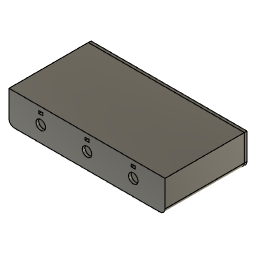
Massive Knob housing - 3 pots, under desk, Arduino Pro Micro (Autodesk Fusion 360 design; units mm, degrees)
Autodesk Fusion 360 part; units mm, degrees
sketch "Housing" plane through (0, 0, 0) normal (0, 1, 0) x (1, 0, 0) in component "Housing"
  line L0 (0, 0) -> (118, 0)
  circle A0 centre (24, -12) radius 3.6
  line L1 (24, -12) -> (24, -20.75) construction
  line L2 (25.5, -20.75) -> (22.5, -20.75)
  line L3 (22.5, -20.75) -> (22.5, -18.75)
  line L4 (22.5, -18.75) -> (25.5, -18.75)
  line L5 (25.5, -18.75) -> (25.5, -20.75)
  circle A1 centre (24, -12) radius 10 construction
  line L6 (24, -12) -> (59, -12) construction
  line L7 (59, -12) -> (94, -12) construction
  circle A2 centre (59, -12) radius 3.6
  circle A3 centre (94, -12) radius 3.6
  line L8 (57.5, -20.75) -> (60.5, -20.75)
  line L9 (60.5, -20.75) -> (60.5, -18.75)
  line L10 (60.5, -18.75) -> (57.5, -18.75)
  line L11 (57.5, -18.75) -> (57.5, -20.75)
  line L12 (92.5, -20.75) -> (95.5, -20.75)
  line L13 (95.5, -20.75) -> (95.5, -18.75)
  line L14 (95.5, -18.75) -> (92.5, -18.75)
  line L15 (92.5, -18.75) -> (92.5, -20.75)
  line L16 (59, -12) -> (59, -20.75) construction
  line L17 (94, -12) -> (94, -20.75) construction
  line L18 (24, -12) -> (24, 0) construction
  line L19 (24, -12) -> (0, -12) construction
  line L20 (94, -12) -> (118, -12) construction
  line L21 (24, -12) -> (24, -24) construction
  line L22 (0, 0) -> (0, -24)
  line L23 (0, -24) -> (118, -24)
  line L24 (118, -24) -> (118, 0)
  line L25 (2, -2) -> (116, -2)
  line L26 (116, -22) -> (116, -2)
  line L27 (2, -22) -> (116, -22)
  line L28 (2, -2) -> (2, -22)
  arc A4 (2, -18) -> (2, -6) centre (2, -12) ccw
  circle A5 centre (3.75, -12) radius 1.75
  arc A6 (116, -6) -> (116, -18) centre (116, -12) ccw
  circle A7 centre (114.25, -12) radius 1.75
  dimension "d1" = 7.2
  dimension "d2" = 8.75
  dimension "d3" = 2
  dimension "d4" = 3
  dimension "d5" = 20
  dimension "d6" = 35
  dimension "d17" = -2
  dimension "d22" = 6
  dimension "d23" = 3.5
  dimension "d24" = 6
  dimension "d25" = 3.5
  dimension "d49" = 24
  dimension "d50" = 12
  constraint coincident L0.start L22.start
  constraint horizontal L0
  constraint coincident A0.centre L1.start
  constraint vertical L1
  constraint horizontal L2
  constraint vertical L3
  constraint horizontal L4
  constraint vertical L5
  constraint midpoint L1.end L2
  constraint concentric A0 A1
  constraint perpendicular L1 L6
  constraint parallel L6 L7
  constraint coincident L6.end L7.start
  constraint coincident L7.end A3.centre
  constraint horizontal L8
  constraint vertical L9
  constraint horizontal L10
  constraint vertical L11
  constraint horizontal L12
  constraint vertical L13
  constraint horizontal L14
  constraint vertical L15
  constraint equal L2 L8
  constraint equal L3 L11
  constraint equal L2 L12
  constraint equal L3 L15
  constraint equal A0 A2
  constraint equal A0 A3
  constraint equal L6 L7
  constraint midpoint L8 L16.end
  constraint midpoint L12 L17.end
  constraint vertical L16
  constraint vertical L17
  constraint equal L1 L16
  constraint equal L1 L17
  constraint coincident L0 L18.end
  constraint perpendicular L0 L18
  constraint perpendicular L1 L19
  constraint perpendicular L17 L20
  constraint perpendicular L19 L21
  constraint perpendicular L19 L22
  constraint perpendicular L22 L23
  constraint perpendicular L0 L24
  constraint coincident L21.end L23
  constraint coincident L19.end L22
  constraint coincident L20.end L24
  constraint coincident L28 A4.end
  constraint midpoint L28 A4.centre
  constraint coincident L19 A5.centre
  constraint coincident A4.centre A5
  constraint coincident L26 A6.start
  constraint midpoint L26 A6.centre
  constraint coincident L20 A7.centre
  constraint coincident A6.centre A7
  constraint equal L19 L20
  constraint equal L18 L21
  measures "d1" diameter of A0
  measures "d2" distance of A0.centre L1.end
  measures "d3" distance of L2.start L4.end
  measures "d4" distance of L2.start L2.end
  measures "d5" diameter of A1
  measures "d6" distance of A0.centre L6.end
  measures "d22" radius of A4
  measures "d23" diameter of A5
  measures "d24" distance of A6.centre A6.start
  measures "d25" diameter of A7
  measures "d49" distance of A0.centre L19.end
  measures "d50" distance of A0.centre L21.end
extrude "Extrude1" add sketch "Housing" along normal blind 2 contours L25 L26 L27 L28 A4 A6 | A5 | L28 A4 | A7 | L26 A6 makes body 1 in component "Housing"
extrude "Extrude3" add sketch "Housing" along normal blind 60 contours L0 L22 L23 L24 bodies 1 in component "Housing"
extrude "Extrude4" add sketch "Housing" against normal blind 5 from surface at 60 contours L28 A4 | L26 A6 bodies 1 in component "Housing"
extrude "Extrude5" add sketch "Housing" against normal blind 2 from surface at 55 contours A5 | L28 A4 | A7 | L26 A6 bodies 1 in component "Housing"
fillet "Fillet1" radius 4 4 edges at (116, 31, 2) (2, 31, 2) (118, 30, 0) (0, 30, 0) on bodies 1 in component "Housing"
chamfer "Chamfer1" distance 5.99 angle 45 2 edges at (2, 53, 12) (116, 53, 12) on bodies 1 in component "Housing"
ref_plane "WorkPlane1" through (0, 60, 0) normal (0, 1, 0) x (0, 0, 1) in component "Lid"
sketch "Lid" plane through (0, 60, 0) normal (0, 1, 0) x (1, 0, 0) in component "Lid"
  arc A0 (6, -2) -> (2, -6) centre (6, -6) ccw construction
  arc A1 (2, -18) -> (2, -6) centre (2, -12) ccw construction
  line L0 (2, -22) -> (2, -18) construction
  line L1 (116, -22) -> (2, -22) construction
  line L2 (6, -2) -> (112, -2) construction
  arc A2 (116, -6) -> (112, -2) centre (112, -6) ccw construction
  arc A3 (116, -6) -> (116, -18) centre (116, -12) ccw construction
  line L3 (116, -18) -> (116, -22) construction
  circle A4 centre (114.25, -12) radius 1.75 construction
  circle A5 centre (3.75, -12) radius 1.75 construction
  circle A6 centre (114.25, -12) radius 1.5
  circle A7 centre (3.75, -12) radius 1.5
  line L4 (0, -24) -> (118, -24)
  line L5 (0, -4) -> (0, -24)
  arc A8 (4, 0) -> (0, -4) centre (4, -4) ccw
  line L6 (114, 0) -> (4, 0)
  arc A9 (118, -4) -> (114, 0) centre (114, -4) ccw
  line L7 (118, -24) -> (118, -4)
  arc A10 (6, -2.4) -> (2.4208, -5.6138) centre (6, -6) ccw
  arc A11 (2.4, -18.3875) -> (2.4208, -5.6138) centre (2, -12) ccw
  line L8 (2.4, -21.6) -> (2.4, -18.3875)
  line L9 (115.6, -21.6) -> (2.4, -21.6)
  line L10 (115.6, -18.3875) -> (115.6, -21.6)
  arc A12 (115.5792, -5.6138) -> (115.6, -18.3875) centre (116, -12) ccw
  arc A13 (115.5792, -5.6138) -> (112, -2.4) centre (112, -6) ccw
  line L11 (6, -2.4) -> (112, -2.4)
  arc A14 (6, -4.4) -> (5.6561, -4.4374) centre (6, -6) ccw
  arc A15 (5.5777, -19.6) -> (5.6561, -4.4374) centre (2, -12) ccw
  line L12 (112.4223, -19.6) -> (5.5777, -19.6)
  arc A16 (112.3439, -4.4374) -> (112.4223, -19.6) centre (116, -12) ccw
  arc A17 (112.3439, -4.4374) -> (112, -4.4) centre (112, -6) ccw
  line L13 (6, -4.4) -> (112, -4.4)
  dimension "d51" = 3
  dimension "d52" = 3
  dimension "d53" = 0.4
  dimension "d54" = 2.4
  constraint concentric A4 A6
  constraint concentric A5 A7
  measures "d51" diameter of A6
  measures "d52" diameter of A7
extrude "Extrude1'" add sketch "Lid" along normal blind 2 separate body contours L4 L5 A8 L6 A9 L7 | A10 A11 L8 L9 L10 A12 A13 L11 | A14 A15 L12 A16 A17 L13 makes body 2 in component "Lid"
extrude "Extrude2" add sketch "Lid" against normal blind 2 contours A10 A11 L8 L9 L10 A12 A13 L11 bodies 2 in component "Lid"
sketch "Arduino Pro Micro USB port" plane through (0, 0, 0) normal (-1, 0, 0) x (0, -1, 0) in component "Housing"
  line L0 (-60, 4) -> (0, 4)
  line L1 (0, 4) -> (0, 24)
  line L2 (0, 24) -> (-60, 24)
  line L3 (-60, 24) -> (-60, 4)
  line L4 (-2, 22) -> (-60, 22)
  line L5 (-31, 22) -> (-31, 19) construction
  line L6 (-35, 19) -> (-27, 19)
  line L7 (-27, 19) -> (-27, 16)
  line L8 (-27, 16) -> (-35, 16)
  line L9 (-35, 16) -> (-35, 19)
  dimension "d43" = 3
  dimension "d44" = 8
  dimension "d45" = 3
  constraint midpoint L4 L5.start
  constraint perpendicular L4 L5
  constraint horizontal L6
  constraint vertical L7
  constraint horizontal L8
  constraint vertical L9
  constraint midpoint L5.end L6
  measures "d43" distance of L5.start L5.end
  measures "d44" distance of L6.start L6.end
  measures "d45" distance of L6.start L8.end
extrude "Extrude6" cut sketch "Arduino Pro Micro USB port" against normal blind 2 contours L6 L7 L8 L9 bodies 1 in component "Housing"
chamfer "Chamfer2" distance 1 angle 45 2 edges at (1, 27, 19) (1, 35, 19) on bodies 1 in component "Housing"
sketch "Arduino Pro Micro support" plane through (0, 0, 22) normal (0, 0, -1) x (1, 0, 0) in component "Housing"
  line L0 (116, -2) -> (2, -2)
  line L1 (2, -2) -> (2, -60)
  line L2 (2, -60) -> (116, -60)
  line L3 (116, -60) -> (116, -2)
  line L4 (2, -2) -> (2, -60)
  line L5 (2, -31) -> (35.5, -31) construction
  line L6 (37.5, -36) -> (35.5, -36)
  line L7 (35.5, -36) -> (35.5, -26)
  line L8 (35.5, -26) -> (37.5, -26)
  line L9 (37.5, -26) -> (37.5, -36)
  dimension "d55" = 33.5
  dimension "d56" = 2
  dimension "d57" = 10
  constraint midpoint L4 L5.start
  constraint perpendicular L1 L5
  constraint horizontal L6
  constraint vertical L7
  constraint horizontal L8
  constraint vertical L9
  constraint midpoint L5.end L7
  measures "d55" distance of L5.start L5.end
  measures "d56" distance of L6.start L6.end
  measures "d57" distance of L6.start L8.end
extrude "Extrude7" add sketch "Arduino Pro Micro support" along normal blind 5 contours L6 L7 L8 L9 bodies 1 in component "Housing"
chamfer "Chamfer3" distance 5 angle 45 2 edges at (36.5, 36, 22) (36.5, 26, 22) on bodies 1 in component "Housing"
chamfer "Chamfer4" distance 5 angle 45 1 edges at (37.5, 31, 22) on bodies 1 in component "Housing"
component "Housing" placed x (1, 0, 0) y (0, 1, 0) z (0, 0, 1) at (0, 0, 0)
component "Lid" placed x (1, 0, 0) y (0, 1, 0) z (0, 0, 1) at (0, 0, 0)
equation "d2 = ( 17.5 / 2 ) * 1 mm"
equation "d24 = d22"
equation "d25 = d23"
equation "d49 = d5 + 4 mm"
named bodies: "Housing", "Lid"
